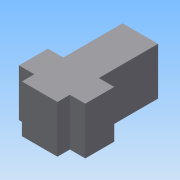
# Autodesk Inventor part: крепеж  для бокса
Saved by Autodesk Inventor 2017 (Build 210142000, 142)
## iProperties
Part Number: крепеж  для бокса
Material: Типовые
Document SubType Name: Modeling
Designer: Max
Mass: 0.64474 g
Surface Area: 6.51926 cm^2
Volume: 0.64474 cm^3
Density: 1 g/cm^3
Appearance: Резина — синяя
Author: Max
Autodesk Inventor part; units mm, degrees
(part 1 of 2)
ref_plane "YZ Plane" through (0, 0, 0) normal (1, 0, 0) x (0, 1, 0)
ref_plane "XZ Plane" through (0, 0, 0) normal (0, 1, 0) x (-1, 0, 0)
ref_plane "XY Plane" through (0, 0, 0) normal (0, 0, 1) x (1, 0, 0)
sketch "Эскиз1" plane through (0, 0, 0) normal (0, 0, 1) x (1, 0, 0)
  line L0 (330.6864, -227.7379) -> (330.6864, -232.7379)
  line L1 (330.6864, -232.7379) -> (331.9864, -232.7379)
  line L2 (331.9864, -232.7379) -> (331.9864, -235.1879)
  line L3 (331.9864, -235.1879) -> (330.6864, -235.1879)
  line L4 (330.6864, -235.1879) -> (330.6864, -236.2379)
  line L5 (330.6864, -236.2379) -> (327.6864, -236.2379)
  line L6 (327.6864, -236.2379) -> (327.6864, -235.1879)
  line L7 (327.6864, -235.1879) -> (326.3864, -235.1879)
  line L8 (326.3864, -235.1879) -> (326.3864, -232.7379)
  line L9 (326.3864, -232.7379) -> (327.6864, -232.7379)
  line L10 (327.6864, -232.7379) -> (327.6864, -227.7379)
  line L11 (327.6864, -227.7379) -> (289.8864, -227.7379)
  line L12 (289.8864, -227.7379) -> (289.8864, -223.7379)
  line L13 (289.8864, -223.7379) -> (212.4864, -223.7379)
  line L14 (212.4864, -223.7379) -> (212.4864, -227.7379)
  line L15 (212.4864, -227.7379) -> (174.8364, -227.7379)
  line L16 (174.8364, -227.7379) -> (174.8364, -232.7379)
  line L17 (174.8364, -232.7379) -> (176.1364, -232.7379)
  line L18 (176.1364, -232.7379) -> (176.1364, -235.1879)
  line L19 (176.1364, -235.1879) -> (174.8364, -235.1879)
  line L20 (174.8364, -235.1879) -> (174.8364, -236.2379)
  line L21 (174.8364, -236.2379) -> (171.8364, -236.2379)
  line L22 (171.8364, -236.2379) -> (171.8364, -235.1879)
  line L23 (171.8364, -235.1879) -> (170.5364, -235.1879)
  line L24 (170.5364, -235.1879) -> (170.5364, -232.7379)
  line L25 (170.5364, -232.7379) -> (171.8364, -232.7379)
  line L26 (171.8364, -232.7379) -> (171.8364, -227.7379)
  line L27 (171.8364, -227.7379) -> (134.1864, -227.7379)
  line L28 (134.1864, -227.7379) -> (134.1864, -735.7379) projected
  line L29 (134.1864, -735.7379) -> (184.1864, -735.7379) projected
  line L30 (184.1864, -735.7379) -> (184.1864, -437.7379) projected
  line L31 (184.1864, -437.7379) -> (204.1864, -417.7379)
  line L32 (204.1864, -417.7379) -> (454.1864, -417.7379)
  line L33 (454.1864, -417.7379) -> (474.1864, -437.7379)
  line L34 (474.1864, -437.7379) -> (474.1864, -735.7379) projected
  line L35 (474.1864, -735.7379) -> (524.1864, -735.7379) projected
  line L36 (524.1864, -735.7379) -> (524.1864, -227.7379) projected
  line L37 (524.1864, -227.7379) -> (486.5364, -227.7379)
  line L38 (486.5364, -227.7379) -> (486.5364, -232.7379)
  line L39 (486.5364, -232.7379) -> (487.8364, -232.7379)
  line L40 (487.8364, -232.7379) -> (487.8364, -235.1879)
  line L41 (487.8364, -235.1879) -> (486.5364, -235.1879)
  line L42 (486.5364, -235.1879) -> (486.5364, -236.2379)
  line L43 (486.5364, -236.2379) -> (483.5364, -236.2379)
  line L44 (483.5364, -236.2379) -> (483.5364, -235.1879)
  line L45 (483.5364, -235.1879) -> (482.2364, -235.1879)
  line L46 (482.2364, -235.1879) -> (482.2364, -232.7379)
  line L47 (482.2364, -232.7379) -> (483.5364, -232.7379)
  line L48 (483.5364, -232.7379) -> (483.5364, -227.7379)
  line L49 (483.5364, -227.7379) -> (445.8864, -227.7379)
  line L50 (445.8864, -227.7379) -> (445.8864, -223.7379)
  line L51 (445.8864, -223.7379) -> (368.4864, -223.7379)
  line L52 (368.4864, -223.7379) -> (368.4864, -227.7379)
  line L53 (368.4864, -227.7379) -> (330.6864, -227.7379)
  circle A0 centre (510.1864, -385.7379) radius 5
  circle A1 centre (148.1864, -385.7379) radius 5
  circle A2 centre (150.1864, -412.7379) radius 5
  circle A3 centre (508.1864, -412.7379) radius 5
  line L54 (198.0365, -283.9874) -> (198.0365, -274.4874)
  arc A4 (198.2865, -274.2374) -> (198.0365, -274.4874) centre (198.2865, -274.4874) ccw
  line L55 (198.2865, -274.2374) -> (220.2865, -274.2374)
  arc A5 (220.5365, -274.4874) -> (220.2865, -274.2374) centre (220.2865, -274.4874) ccw
  line L56 (220.5365, -274.4874) -> (220.5365, -283.9874)
  arc A6 (220.2865, -284.2374) -> (220.5365, -283.9874) centre (220.2865, -283.9874) ccw
  line L57 (220.2865, -284.2374) -> (198.2865, -284.2374)
  arc A7 (198.0365, -283.9874) -> (198.2865, -284.2374) centre (198.2865, -283.9874) ccw
  spline S0 degree 4 poles (220.5005, -310.507) (220.5003, -310.0397) (220.4543, -309.4219) (220.3063, -308.6946) (219.9828, -307.9126) (219.5846, -307.2407) (219.1485, -306.7849) (218.7486, -306.4926) (218.4341, -306.3133) knots 0 0 0 0 0 0.333261 0.458786 0.580687 0.70052 1 1 1 1 1
  spline S1 degree 4 poles (218.4341, -306.3133) (218.2194, -306.2045) (217.9574, -306.0638) (217.2245, -305.8515) (216.8112, -305.759) (215.0952, -305.8521) (214.8239, -305.815) knots 0 0 0 0 0 0.331948 0.48487 1 1 1 1 1
  line L58 (214.8239, -305.815) -> (210.9827, -305.815)
  line L59 (210.9827, -305.815) -> (210.9827, -303.0192)
  line L60 (210.9827, -303.0192) -> (215.6262, -303.0192)
  spline S2 degree 4 poles (215.6262, -303.0192) (216.0632, -302.9791) (218.3041, -303.1205) (219.1074, -303.2602) (220.3376, -303.6977) (220.8048, -303.9727) (221.1813, -304.1983) knots 0 0 0 0 0 0.48869 0.646796 1 1 1 1 1
  spline S3 degree 4 poles (221.1813, -304.1983) (221.6328, -304.4905) (222.2206, -304.9662) (222.87, -305.6808) (223.5166, -306.727) (224.0456, -307.8865) (224.2868, -308.9631) (224.3652, -309.8569) (224.366, -310.5313) knots 0 0 0 0 0 0.30127 0.423004 0.546367 0.672176 1 1 1 1 1
  spline S4 degree 4 poles (224.366, -310.5313) (224.3672, -311.1836) (224.2819, -312.0637) (224.0275, -313.128) (223.4629, -314.3083) (222.7851, -315.3791) (222.1412, -316.0885) (221.5656, -316.5539) (221.1326, -316.8279) knots 0 0 0 0 0 0.325829 0.453052 0.578284 0.70143 1 1 1 1 1
  spline S5 degree 4 poles (221.1326, -316.8279) (220.7893, -317.0305) (220.3484, -317.2658) (219.1646, -317.6777) (218.3558, -317.7448) (216.0857, -318.1145) (215.6748, -318.0192) knots 0 0 0 0 0 0.345082 0.503845 1 1 1 1 1
  line L61 (215.6748, -318.0192) -> (210.9827, -318.0192)
  line L62 (210.9827, -318.0192) -> (210.9827, -315.2112)
  line L63 (210.9827, -315.2112) -> (214.8239, -315.2112)
  spline S6 degree 4 poles (214.8239, -315.2112) (215.1741, -315.246) (216.9237, -315.0068) (217.3918, -315.0434) (218.1403, -314.8454) (218.4072, -314.7315) (218.6164, -314.6278) knots 0 0 0 0 0 0.523746 0.675711 1 1 1 1 1
  spline S7 degree 4 poles (218.6164, -314.6278) (218.8947, -314.4519) (219.2518, -314.164) (219.6429, -313.721) (220.0126, -313.068) (220.3184, -312.3077) (220.4565, -311.5867) (220.5004, -310.9747) (220.5005, -310.507) knots 0 0 0 0 0 0.293933 0.413176 0.535292 0.661734 1 1 1 1 1
  line L64 (206.7865, -285.7374) -> (206.7865, -284.7374)
  line L65 (206.7865, -284.7374) -> (211.7865, -284.7374)
  line L66 (211.7865, -284.7374) -> (211.7865, -285.7374)
  line L67 (211.7865, -285.7374) -> (213.7865, -285.7374)
  line L68 (213.7865, -285.7374) -> (213.7865, -288.7374)
  spline S8 degree 4 poles (213.7865, -288.7374) (213.6519, -288.8139) (213.4737, -288.7819) (213.3015, -288.643) (213.0567, -288.4771) (212.69, -288.3556) (212.2603, -288.4723) (211.871, -288.6284) (211.5365, -288.7374) knots 0 0 0 0 0 0.262205 0.367936 0.481015 0.607227 1 1 1 1 1
  spline S9 degree 4 poles (211.5365, -288.7374) (211.1505, -288.9432) (210.6435, -289.1648) (210.0259, -289.3413) (209.2886, -289.3933) (208.5507, -289.3412) (207.9319, -289.1646) (207.4237, -288.9431) (207.0365, -288.7374) knots 0 0 0 0 0 0.321352 0.440904 0.558717 0.678328 1 1 1 1 1
  spline S10 degree 4 poles (207.0365, -288.7374) (206.8474, -288.9124) (206.596, -289.091) (206.2892, -289.2192) (205.9233, -289.2608) (205.553, -289.2318) (205.2381, -289.1011) (204.981, -288.9152) (204.7865, -288.7374) knots 0 0 0 0 0 0.325734 0.441296 0.554264 0.670467 1 1 1 1 1
  line L69 (204.7865, -288.7374) -> (204.7865, -285.7374)
  line L70 (204.7865, -285.7374) -> (206.7865, -285.7374)
  line L71 (209.6615, -293.1605) -> (208.9115, -293.1605)
  line L72 (208.9115, -293.1605) -> (205.8815, -289.9115)
  spline S11 degree 4 poles (205.8815, -289.9115) (205.9805, -289.9087) (206.1201, -289.8928) (206.2986, -289.8511) (206.5123, -289.7699) (206.7297, -289.6659) (206.9037, -289.5566) (207.0382, -289.4574) (207.1348, -289.3787) knots 0 0 0 0 0 0.300687 0.4228 0.546613 0.672716 1 1 1 1 1
  spline S12 degree 4 poles (207.1348, -289.3787) (207.4869, -289.5458) (207.9624, -289.7299) (208.5607, -289.88) (209.2865, -289.9251) (210.0123, -289.88) (210.6106, -289.7298) (211.0863, -289.5458) (211.4383, -289.3787) knots 0 0 0 0 0 0.318028 0.439699 0.56029 0.681964 1 1 1 1 1
  spline S13 degree 4 poles (211.4383, -289.3787) (211.5621, -289.4198) (211.726, -289.4782) (211.9234, -289.5547) (212.1488, -289.6486) (212.3519, -289.7369) (212.5071, -289.8094) (212.6189, -289.8675) (212.6916, -289.9115) knots 0 0 0 0 0 0.337221 0.465736 0.590517 0.711668 1 1 1 1 1
  line L73 (212.6916, -289.9115) -> (209.6615, -293.1605)
  line L74 (214.751, -315.1701) -> (210.9827, -315.1701)
  line L75 (210.9827, -315.1701) -> (210.9827, -305.8193)
  line L76 (210.9827, -305.8193) -> (214.751, -305.8193)
  line L77 (214.751, -305.8193) -> (214.751, -315.1701)
  arc A8 (209.7865, -300.4106) -> (208.2865, -298.9106) centre (208.2865, -300.4106) ccw
  line L78 (209.7865, -300.4106) -> (209.7865, -300.9106)
  line L79 (209.7865, -300.9106) -> (208.7865, -300.9106)
  line L80 (208.7865, -300.9106) -> (208.7865, -300.4106)
  arc A9 (208.7865, -300.4106) -> (208.2865, -299.9106) centre (208.2865, -300.4106) ccw
  line L81 (208.2865, -299.9106) -> (201.7865, -299.9106)
  arc A10 (201.7865, -296.9106) -> (201.7865, -299.9106) centre (201.7865, -298.4106) ccw
  line L82 (201.7865, -296.9106) -> (216.7865, -296.9106)
  arc A11 (216.7865, -296.9106) -> (216.7865, -295.9106) centre (216.7865, -296.4106) ccw
  line L83 (216.7865, -295.9106) -> (210.2865, -295.9106)
  arc A12 (208.7865, -294.4106) -> (210.2865, -295.9106) centre (210.2865, -294.4106) ccw
  line L84 (208.7865, -294.4106) -> (208.7865, -293.9106)
  line L85 (208.7865, -293.9106) -> (209.7865, -293.9106)
  line L86 (209.7865, -293.9106) -> (209.7865, -294.4106)
  arc A13 (209.7865, -294.4106) -> (210.2865, -294.9106) centre (210.2865, -294.4106) ccw
  line L87 (210.2865, -294.9106) -> (216.7865, -294.9106)
  arc A14 (216.7865, -297.9106) -> (216.7865, -294.9106) centre (216.7865, -296.4106) ccw
  line L88 (216.7865, -297.9106) -> (201.7865, -297.9106)
  arc A15 (201.7865, -297.9106) -> (201.7865, -298.9106) centre (201.7865, -298.4106) ccw
  line L89 (201.7865, -298.9106) -> (208.2865, -298.9106)
  spline S14 degree 4 poles (206.5338, -303.6148) (206.7685, -303.7597) (207.0659, -303.9867) (207.3902, -304.3236) (207.6872, -304.8028) (207.9226, -305.3279) (208.031, -305.7914) (208.0657, -306.1761) (208.0654, -306.4592) knots 0 0 0 0 0 0.312949 0.435922 0.558791 0.682637 1 1 1 1 1
  spline S15 degree 4 poles (208.0654, -306.4592) (208.0667, -306.8455) (207.9969, -307.373) (207.7865, -307.9991) (207.3334, -308.6976) (206.7816, -309.3133) (206.2308, -309.6699) (205.74, -309.8607) (205.3668, -309.9479) knots 0 0 0 0 0 0.313918 0.438715 0.563217 0.687663 1 1 1 1 1
  line L90 (205.3668, -309.9479) -> (205.3668, -310.0937)
  spline S16 degree 4 poles (205.3668, -310.0937) (205.5312, -310.0712) (206.2732, -310.3709) (206.5855, -310.4525) (207.0618, -310.7261) (207.2515, -310.8673) (207.409, -310.9933) knots 0 0 0 0 0 0.467412 0.627499 1 1 1 1 1
  spline S17 degree 4 poles (207.409, -310.9933) (207.5481, -311.1133) (207.7331, -311.307) (207.9398, -311.5886) (208.1607, -311.9975) (208.3429, -312.4401) (208.4267, -312.8625) (208.4538, -313.2077) (208.4544, -313.473) knots 0 0 0 0 0 0.293401 0.414689 0.538726 0.665972 1 1 1 1 1
  spline S18 degree 4 poles (208.4544, -313.473) (208.4542, -313.8182) (208.4167, -314.2867) (208.3007, -314.8566) (208.0496, -315.5046) (207.7363, -316.1003) (207.4002, -316.53) (207.0921, -316.8283) (206.8498, -317.0224) knots 0 0 0 0 0 0.321122 0.446176 0.569734 0.692519 1 1 1 1 1
  spline S19 degree 4 poles (206.8498, -317.0224) (206.6091, -317.215) (206.2427, -317.4621) (205.7289, -317.7312) (205.0243, -317.9925) (204.2362, -318.2079) (203.4791, -318.3046) (202.8516, -318.3351) (202.3644, -318.3352) knots 0 0 0 0 0 0.288505 0.407246 0.52959 0.656869 1 1 1 1 1
  spline S20 degree 4 poles (202.3644, -318.3352) (200.7651, -318.3047) (199.5638, -318.1496) (198.2039, -317.74) (197.3198, -317.3871) knots 0 0 0 0 0 1 1 1 1 1
  line L91 (197.3198, -317.3871) -> (197.3198, -314.1294)
  line L92 (197.3198, -314.1294) -> (197.6845, -314.1294)
  spline S21 degree 4 poles (197.6845, -314.1294) (197.8963, -314.3375) (199.3348, -314.8985) (200.0458, -315.1512) (200.9862, -315.3661) (201.3735, -315.4088) (201.6594, -315.43) knots 0 0 0 0 0 0.485606 0.650571 1 1 1 1 1
  spline S22 degree 4 poles (201.6594, -315.43) (201.8017, -315.4566) (202.7287, -315.3618) (203.1091, -315.3075) (203.6053, -315.1248) (203.7864, -315.012) (203.9203, -314.9195) knots 0 0 0 0 0 0.490597 0.653392 1 1 1 1 1
  spline S23 degree 4 poles (203.9203, -314.9195) (204.0251, -314.8403) (204.1632, -314.7177) (204.3146, -314.5417) (204.4732, -314.2933) (204.5993, -314.0182) (204.6569, -313.7148) (204.6734, -313.4623) (204.674, -313.2542) knots 0 0 0 0 0 0.293695 0.410721 0.530018 0.654429 1 1 1 1 1
  spline S24 degree 4 poles (204.674, -313.2542) (204.6737, -313.05) (204.65, -312.7949) (204.5704, -312.5) (204.3941, -312.2275) (204.1685, -311.9914) (203.9524, -311.8427) (203.754, -311.7508) (203.6043, -311.6983) knots 0 0 0 0 0 0.332874 0.455336 0.574642 0.693712 1 1 1 1 1
  spline S25 degree 3 poles (203.6043, -311.6983) (203.1339, -311.419) (202.8478, -311.2752) (201.2461, -311.4916) knots 0 0 0 0 1 1 1 1
  line L93 (201.2461, -311.4916) -> (200.6018, -311.4916)
  line L94 (200.6018, -311.4916) -> (200.6018, -308.8539)
  line L95 (200.6018, -308.8539) -> (201.1975, -308.8539)
  spline S26 degree 4 poles (201.1975, -308.8539) (201.8646, -308.8347) (202.5816, -308.7738) (203.0974, -308.7347) (203.4341, -308.55) knots 0 0 0 0 0 1 1 1 1 1
  spline S27 degree 4 poles (203.4341, -308.55) (203.5568, -308.4899) (203.7161, -308.3919) (203.8905, -308.2415) (204.0639, -308.0177) (204.2017, -307.7644) (204.265, -307.4981) (204.2843, -307.2719) (204.285, -307.0913) knots 0 0 0 0 0 0.303428 0.422137 0.541736 0.664935 1 1 1 1 1
  spline S28 degree 4 poles (204.285, -307.0913) (204.2846, -306.9506) (204.2677, -306.7719) (204.2092, -306.5582) (204.0845, -306.3506) (203.9226, -306.1579) (203.7804, -306.033) (203.6505, -305.9492) (203.5557, -305.9001) knots 0 0 0 0 0 0.328861 0.453441 0.575803 0.697309 1 1 1 1 1
  spline S29 degree 4 poles (203.5557, -305.9001) (203.4448, -305.8495) (203.2969, -305.7896) (202.9114, -305.6871) (202.6272, -305.6603) (201.9555, -305.5746) (201.8782, -305.5962) knots 0 0 0 0 0 0.352064 0.518119 1 1 1 1 1
  spline S30 degree 4 poles (201.8782, -305.5962) (201.3241, -305.5966) (200.7829, -305.6848) (200.1681, -305.8558) (199.6416, -306.0581) knots 0 0 0 0 0 1 1 1 1 1
  spline S31 degree 3 poles (199.6416, -306.0581) (200.0559, -305.6978) (203.2118, -303.6988) (198.2887, -306.7332) knots 0 0 0 0 1 1 1 1
  line L96 (198.2887, -306.7332) -> (197.8235, -306.8604)
  line L97 (197.8235, -306.8604) -> (197.7574, -306.8604)
  line L98 (197.7574, -306.8604) -> (197.7574, -303.6513)
  spline S32 degree 4 poles (197.7574, -303.6513) (198.6005, -303.3178) (200.0612, -302.9118) (201.2135, -302.7136) (202.5346, -302.7031) knots 0 0 0 0 0 1 1 1 1 1
  spline S33 degree 4 poles (202.5346, -302.7031) (203.7734, -302.7074) (204.8441, -302.8363) (205.7919, -303.1378) (206.5338, -303.6148) knots 0 0 0 0 0 1 1 1 1 1
  line L99 (209.1913, -331.2373) -> (209.1913, -324.7373)
  arc A16 (209.1913, -324.7373) -> (209.1912, -324.7373) centre (209.2865, -297.2374) ccw
  line L100 (209.1912, -324.7373) -> (209.1912, -331.2373)
  arc A17 (204.7865, -330.9383) -> (209.1912, -331.2373) centre (209.2865, -297.2374) ccw
  arc A18 (203.0365, -327.6009) -> (204.7865, -330.9383) centre (216.5671, -322.6337) ccw
  arc A19 (192.2358, -323.127) -> (203.0365, -327.6009) centre (209.2865, -297.2374) ccw
  arc A20 (188.6384, -324.2495) -> (192.2358, -323.127) centre (186.1806, -310.0472) ccw
  arc A21 (182.2744, -317.8856) -> (188.6384, -324.2495) centre (209.2865, -297.2374) ccw
  arc A22 (183.3969, -314.2882) -> (182.2744, -317.8856) centre (196.4768, -320.3434) ccw
  arc A23 (178.9231, -303.4874) -> (183.3969, -314.2882) centre (209.2865, -297.2374) ccw
  arc A24 (175.5856, -301.7374) -> (178.9231, -303.4874) centre (183.8903, -289.9569) ccw
  arc A25 (175.5856, -292.7374) -> (175.5856, -301.7374) centre (209.2865, -297.2374) ccw
  arc A26 (178.9231, -290.9874) -> (175.5856, -292.7374) centre (183.8903, -304.518) ccw
  arc A27 (183.3969, -280.1867) -> (178.9231, -290.9874) centre (209.2865, -297.2374) ccw
  arc A28 (182.2744, -276.5893) -> (183.3969, -280.1867) centre (196.4768, -274.1315) ccw
  arc A29 (188.6384, -270.2253) -> (182.2744, -276.5893) centre (209.2865, -297.2374) ccw
  arc A30 (192.2358, -271.3478) -> (188.6384, -270.2253) centre (186.1806, -284.4277) ccw
  arc A31 (203.0365, -266.874) -> (192.2358, -271.3478) centre (209.2865, -297.2374) ccw
  arc A32 (204.7865, -263.5365) -> (203.0365, -266.874) centre (216.5671, -271.8412) ccw
  arc A33 (213.7865, -263.5365) -> (204.7865, -263.5365) centre (209.2865, -297.2374) ccw
  arc A34 (215.5365, -266.874) -> (213.7865, -263.5365) centre (202.006, -271.8412) ccw
  arc A35 (226.3373, -271.3478) -> (215.5365, -266.874) centre (209.2865, -297.2374) ccw
  arc A36 (229.9347, -270.2253) -> (226.3373, -271.3478) centre (232.3925, -284.4277) ccw
  arc A37 (236.2986, -276.5893) -> (229.9347, -270.2253) centre (209.2865, -297.2374) ccw
  arc A38 (235.1761, -280.1867) -> (236.2986, -276.5893) centre (222.0963, -274.1315) ccw
  arc A39 (239.65, -290.9874) -> (235.1761, -280.1867) centre (209.2865, -297.2374) ccw
  arc A40 (242.9874, -292.7374) -> (239.65, -290.9874) centre (234.6828, -304.518) ccw
  arc A41 (242.9874, -301.7374) -> (242.9874, -292.7374) centre (209.2865, -297.2374) ccw
  arc A42 (239.65, -303.4874) -> (242.9874, -301.7374) centre (234.6828, -289.9569) ccw
  arc A43 (235.1761, -314.2882) -> (239.65, -303.4874) centre (209.2865, -297.2374) ccw
  arc A44 (236.2986, -317.8856) -> (235.1761, -314.2882) centre (222.0963, -320.3434) ccw
  arc A45 (229.9347, -324.2495) -> (236.2986, -317.8856) centre (209.2865, -297.2374) ccw
  arc A46 (226.3373, -323.127) -> (229.9347, -324.2495) centre (232.3925, -310.0472) ccw
  arc A47 (215.5365, -327.6009) -> (226.3373, -323.127) centre (209.2865, -297.2374) ccw
  arc A48 (213.7865, -330.9383) -> (215.5365, -327.6009) centre (202.006, -322.6337) ccw
  arc A49 (209.1913, -331.2373) -> (213.7865, -330.9383) centre (209.2865, -297.2374) ccw
  circle A50 centre (330.1864, -297.7379) radius 20.6
  circle A51 centre (508.6864, -721.7379) radius 2 projected
  circle A52 centre (149.6864, -682.2379) radius 2 projected
  circle A53 centre (149.6864, -424.7379) radius 2
  circle A54 centre (508.6864, -424.7379) radius 2
  circle A55 centre (508.6864, -506.7379) radius 2.875 projected
  circle A56 centre (149.6864, -453.7379) radius 2
  circle A57 centre (149.6864, -721.7379) radius 2 projected
  circle A58 centre (170.4364, -639.7379) radius 1.5 projected
  circle A59 centre (170.4364, -507.7379) radius 1.5 projected
  circle A60 centre (170.4364, -477.7379) radius 1.5
  circle A61 centre (170.4364, -669.7379) radius 1.5 projected
  circle A62 centre (479.4534, -583.2596) radius 1.5 projected
  line L101 (445.4108, -378.2955) -> (445.4108, -381.1733)
  line L102 (445.4108, -381.1733) -> (439.6177, -381.1733)
  line L103 (439.6177, -381.1733) -> (439.3174, -383.1252)
  spline S34 degree 4 poles (439.3174, -383.1252) (439.8832, -382.9763) (440.4727, -382.8362) (441.0568, -382.6943) (441.6697, -382.5621) knots 0 0 0 0 0 1 1 1 1 1
  spline S35 degree 4 poles (441.6697, -382.5621) (442.2638, -382.5598) (443.052, -382.6679) (443.9476, -382.9985) (444.8569, -383.7336) (445.5947, -384.609) (445.9315, -385.4454) (446.0393, -386.1746) (446.0364, -386.7161) knots 0 0 0 0 0 0.321 0.445325 0.568168 0.690637 1 1 1 1 1
  spline S36 degree 4 poles (446.0364, -386.7161) (446.0346, -387.3159) (445.9109, -388.0809) (445.4981, -389.1528) (444.7052, -390.1668) (443.6543, -391.0177) (442.5576, -391.4124) (441.5087, -391.5161) (440.7063, -391.5207) knots 0 0 0 0 0 0.301808 0.422596 0.543783 0.666952 1 1 1 1 1
  spline S37 degree 4 poles (440.7063, -391.5207) (439.918, -391.5188) (438.9727, -391.4394) (437.9148, -391.1682) (436.9202, -390.5588) (436.1038, -389.8278) (435.6627, -389.1519) (435.3981, -388.4698) (435.2385, -387.9298) knots 0 0 0 0 0 0.344288 0.467767 0.585513 0.701061 1 1 1 1 1
  line L104 (435.2385, -387.9298) -> (438.892, -387.5294)
  spline S38 degree 4 poles (438.892, -387.5294) (438.9412, -387.7989) (439.0435, -388.1412) (439.2278, -388.5159) (439.5476, -388.8668) (439.8937, -389.136) (440.207, -389.2665) (440.4728, -389.3137) (440.6687, -389.3186) knots 0 0 0 0 0 0.337823 0.463732 0.585419 0.704571 1 1 1 1 1
  spline S39 degree 4 poles (440.6687, -389.3186) (440.8901, -389.3188) (441.1893, -389.2693) (441.5319, -389.1156) (441.8931, -388.7807) (442.2105, -388.3375) (442.349, -387.842) (442.3952, -387.3979) (442.3954, -387.0414) knots 0 0 0 0 0 0.288865 0.405011 0.524609 0.650411 1 1 1 1 1
  spline S40 degree 4 poles (442.3954, -387.0414) (442.3965, -386.6796) (442.3506, -386.2306) (442.2143, -385.7358) (441.8934, -385.3038) (441.5184, -384.9825) (441.1547, -384.8384) (440.8338, -384.7976) (440.5936, -384.8018) knots 0 0 0 0 0 0.347295 0.471219 0.589277 0.705046 1 1 1 1 1
  spline S41 degree 4 poles (440.5936, -384.8018) (440.3308, -384.8028) (440.0722, -384.8472) (439.8214, -384.9358) (439.5802, -385.0645) knots 0 0 0 0 0 1 1 1 1 1
  spline S42 degree 4 poles (439.5802, -385.0645) (439.4113, -385.0419) (439.2106, -385.2032) (439.0118, -385.4464) (438.7919, -385.7277) knots 0 0 0 0 0 1 1 1 1 1
  line L105 (438.7919, -385.7277) -> (435.714, -385.2897)
  line L106 (435.714, -385.2897) -> (436.8526, -378.2955)
  line L107 (436.8526, -378.2955) -> (445.4108, -378.2955)
  spline S43 degree 4 poles (406.7861, -386.7537) (406.783, -386.8994) (406.9374, -387.4742) (407.0204, -387.7031) (407.1624, -387.996) (407.2325, -388.1023) (407.2866, -388.18) knots 0 0 0 0 0 0.506296 0.664932 1 1 1 1 1
  spline S44 degree 4 poles (407.2866, -388.18) (407.382, -388.3002) (407.5282, -388.4525) (407.7394, -388.6182) (408.0321, -388.7711) (408.3561, -388.8938) (408.6492, -388.9503) (408.8932, -388.9682) (409.0758, -388.9683) knots 0 0 0 0 0 0.304407 0.425791 0.548382 0.673395 1 1 1 1 1
  spline S45 degree 4 poles (409.0758, -388.9683) (409.3418, -388.9666) (409.6834, -388.9198) (410.0596, -388.803) (410.4185, -388.5341) (410.6892, -388.2467) (410.8181, -387.9944) (410.8631, -387.7819) (410.8651, -387.6295) knots 0 0 0 0 0 0.349494 0.478462 0.601477 0.719585 1 1 1 1 1
  spline S46 degree 4 poles (410.8651, -387.6295) (410.8651, -387.5535) (410.8554, -387.4485) (410.8248, -387.3165) (410.7593, -387.1612) (410.6716, -387.0048) (410.5753, -386.883) (410.4859, -386.792) (410.4146, -386.7286) knots 0 0 0 0 0 0.300852 0.421911 0.544763 0.670489 1 1 1 1 1
  spline S47 degree 4 poles (410.4146, -386.7286) (410.1571, -386.5044) (409.6674, -386.3111) (409.0725, -386.1312) (408.3627, -385.9654) knots 0 0 0 0 0 1 1 1 1 1
  spline S48 degree 4 poles (408.3627, -385.9654) (407.1494, -385.6938) (406.0889, -385.3543) (405.2024, -384.9288) (404.584, -384.3889) knots 0 0 0 0 0 1 1 1 1 1
  spline S49 degree 4 poles (404.584, -384.3889) (404.408, -384.2361) (404.1857, -384.0093) (403.9447, -383.6933) (403.7233, -383.2707) (403.5506, -382.824) (403.4707, -382.4311) (403.4454, -382.1105) (403.4454, -381.874) knots 0 0 0 0 0 0.314239 0.437484 0.560343 0.683894 1 1 1 1 1
  spline S50 degree 4 poles (403.4454, -381.874) (403.4449, -381.4151) (403.5577, -380.8163) (403.9167, -380.0101) (404.6502, -379.2264) (405.7309, -378.5045) (406.8706, -378.1485) (408.0596, -378.0831) (408.9757, -378.0703) knots 0 0 0 0 0 0.276596 0.390848 0.509627 0.635941 1 1 1 1 1
  spline S51 degree 4 poles (408.9757, -378.0703) (409.7519, -378.0735) (410.7314, -378.1522) (411.8268, -378.4191) (412.8553, -379.0125) (413.6516, -379.7584) (414.0771, -380.5932) (414.2667, -381.3518) (414.3434, -381.949) knots 0 0 0 0 0 0.340632 0.462675 0.579541 0.695373 1 1 1 1 1
  line L108 (414.3434, -381.949) -> (410.5523, -382.1743)
  spline S52 degree 4 poles (410.5523, -382.1743) (410.5026, -381.9089) (410.4058, -381.5777) (410.2218, -381.2167) (409.9086, -380.8975) (409.5367, -380.6514) (409.1622, -380.5366) (408.8314, -380.5001) (408.5754, -380.4976) knots 0 0 0 0 0 0.324684 0.444588 0.562205 0.68129 1 1 1 1 1
  spline S53 degree 4 poles (408.5754, -380.4976) (408.3547, -380.4984) (408.0765, -380.531) (407.7733, -380.6151) (407.4955, -380.8115) (407.2908, -381.0256) (407.1945, -381.225) (407.1626, -381.397) (407.1615, -381.5236) knots 0 0 0 0 0 0.354168 0.481315 0.601534 0.717295 1 1 1 1 1
  spline S54 degree 4 poles (407.1615, -381.5236) (407.151, -381.5513) (407.1425, -381.5923) (407.1555, -381.6537) (407.1952, -381.7382) (407.2603, -381.845) (407.3352, -381.9396) (407.4052, -382.0169) (407.4618, -382.0742) knots 0 0 0 0 0 0.247386 0.359721 0.483602 0.619276 1 1 1 1 1
  spline S55 degree 4 poles (407.4618, -382.0742) (407.502, -382.1096) (407.5742, -382.1593) (407.6951, -382.2227) (407.9699, -382.3345) (408.225, -382.4111) (408.4138, -382.46) (408.8131, -382.5496) knots 0 0 0 0 0 0.265093 0.389381 0.526504 1 1 1 1 1
  spline S56 degree 4 poles (408.8131, -382.5496) (409.9591, -382.8033) (411.5127, -383.2002) (412.6708, -383.6431) (413.7254, -384.4472) (414.3811, -385.2229) (414.6765, -385.9927) (414.7705, -386.6006) (414.7688, -387.0665) knots 0 0 0 0 0 0.389595 0.513425 0.625734 0.733468 1 1 1 1 1
  spline S57 degree 4 poles (414.7688, -387.0665) (414.7651, -387.6424) (414.6429, -388.3842) (414.1942, -389.3533) (413.3387, -390.2809) (412.195, -391.0651) (411.0021, -391.4207) (409.8737, -391.5173) (409.0008, -391.5207) knots 0 0 0 0 0 0.292777 0.410851 0.531211 0.655943 1 1 1 1 1
  spline S58 degree 4 poles (409.0008, -391.5207) (407.9895, -391.5206) (406.7811, -391.4067) (405.4293, -391.0713) (404.3652, -390.2519) (403.5782, -389.2777) (403.1749, -388.3819) (403.0083, -387.5819) (402.9575, -386.9914) knots 0 0 0 0 0 0.35491 0.478284 0.59487 0.709037 1 1 1 1 1
  line L109 (402.9575, -386.9914) -> (406.7861, -386.7537)
  spline S59 degree 4 poles (394.7371, -378.0703) (395.7191, -378.07) (396.9898, -378.2189) (398.4153, -378.6999) (399.7793, -379.7808) (400.8604, -381.1289) (401.3447, -382.5175) (401.4939, -383.753) (401.4936, -384.7017) knots 0 0 0 0 0 0.321996 0.442966 0.562085 0.682373 1 1 1 1 1
  spline S60 degree 4 poles (401.4936, -384.7017) (401.4851, -385.7192) (401.3652, -387.0404) (400.8679, -388.4392) (399.8128, -389.7826) (398.4904, -390.8562) (397.1164, -391.3853) (395.8566, -391.5119) (394.8872, -391.5207) knots 0 0 0 0 0 0.324201 0.444012 0.561748 0.68112 1 1 1 1 1
  spline S61 degree 4 poles (394.8872, -391.5207) (393.9051, -391.5237) (392.6153, -391.3825) (391.2354, -390.9616) (389.8902, -389.9369) (388.7595, -388.5767) (388.1566, -387.1369) (388.0342, -385.8227) (388.0181, -384.8018) knots 0 0 0 0 0 0.317732 0.436395 0.554274 0.675018 1 1 1 1 1
  spline S62 degree 4 poles (388.0181, -384.8018) (388.017, -383.8398) (388.1688, -382.5871) (388.6587, -381.1773) (389.7545, -379.8084) (391.1224, -378.7124) (392.5286, -378.2217) (393.7783, -378.0695) (394.7371, -378.0703) knots 0 0 0 0 0 0.319418 0.440426 0.560018 0.68097 1 1 1 1 1
  line L110 (364.7958, -383.8884) -> (371.0017, -383.8884)
  line L111 (371.0017, -383.8884) -> (371.0017, -389.4187)
  spline S63 degree 4 poles (371.0017, -389.4187) (369.2773, -390.5761) (367.9432, -391.1503) (366.483, -391.341) (364.5956, -391.5207) knots 0 0 0 0 0 1 1 1 1 1
  spline S64 degree 4 poles (364.5956, -391.5207) (363.5663, -391.5174) (362.2259, -391.3822) (360.8136, -390.891) (359.4739, -389.7879) (358.4229, -388.4046) (357.8973, -386.926) (357.756, -385.7341) (357.7515, -384.7893) knots 0 0 0 0 0 0.324055 0.444084 0.562865 0.683419 1 1 1 1 1
  spline S65 degree 4 poles (357.7515, -384.7893) (357.7514, -384.1263) (357.8305, -383.2389) (358.08, -382.1878) (358.6262, -381.0385) (359.3014, -380.0325) (360.0273, -379.366) (360.6882, -378.9465) (361.2048, -378.6959) knots 0 0 0 0 0 0.325345 0.450117 0.57259 0.694038 1 1 1 1 1
  spline S66 degree 4 poles (361.2048, -378.6959) (361.9122, -378.363) (362.7618, -378.1622) (363.7151, -378.0709) (364.7582, -378.0703) knots 0 0 0 0 0 1 1 1 1 1
  spline S67 degree 4 poles (364.7582, -378.0703) (365.6777, -378.0749) (366.95, -378.1343) (367.9815, -378.3613) (369.0464, -378.967) (369.8787, -379.6881) (370.3859, -380.4767) (370.6707, -381.1881) (370.8266, -381.7488) knots 0 0 0 0 0 0.355167 0.475286 0.589187 0.703074 1 1 1 1 1
  line L112 (370.8266, -381.7488) -> (366.9478, -382.4495)
  spline S68 degree 4 poles (366.9478, -382.4495) (366.8814, -382.2273) (366.7537, -381.9399) (366.5276, -381.6226) (366.158, -381.3184) (365.7254, -381.0709) (365.3057, -380.9576) (364.9456, -380.9221) (364.6706, -380.923) knots 0 0 0 0 0 0.306162 0.426653 0.548001 0.672045 1 1 1 1 1
  spline S69 degree 4 poles (364.6706, -380.923) (364.2835, -380.9239) (363.7673, -381.0025) (363.1828, -381.2508) (362.5857, -381.7934) (362.0729, -382.5227) (361.8522, -383.3711) (361.781, -384.1317) (361.7804, -384.7517) knots 0 0 0 0 0 0.291183 0.405965 0.523705 0.648116 1 1 1 1 1
  spline S70 degree 4 poles (361.7804, -384.7517) (361.779, -385.4039) (361.8504, -386.201) (362.0651, -387.0776) (362.5841, -387.8163) (363.2003, -388.3522) (363.8218, -388.5952) (364.3751, -388.6679) (364.7958, -388.668) knots 0 0 0 0 0 0.352198 0.4751 0.591203 0.705096 1 1 1 1 1
  spline S71 degree 4 poles (364.7958, -388.668) (365.5044, -388.577) (366.1093, -388.5966) (366.7466, -388.3761) (367.4859, -387.8047) knots 0 0 0 0 0 1 1 1 1 1
  line L113 (367.4859, -387.8047) -> (367.4859, -386.591)
  line L114 (367.4859, -386.591) -> (364.7958, -386.591)
  line L115 (364.7958, -386.591) -> (364.7958, -383.8884)
  line L116 (338.1076, -378.2955) -> (344.8015, -378.2955)
  spline S72 degree 4 poles (344.8015, -378.2955) (345.6091, -378.3087) (346.7113, -378.4377) (347.6525, -378.6374) (348.5774, -379.2274) (349.2936, -379.9502) (349.6937, -380.7224) (349.8093, -381.3789) (349.8314, -381.899) knots 0 0 0 0 0 0.352761 0.473532 0.588688 0.703565 1 1 1 1 1
  spline S73 degree 4 poles (349.8314, -381.899) (349.8301, -382.2318) (349.7876, -382.6715) (349.6583, -383.1996) (349.3774, -383.7638) (349.0247, -384.2843) (348.6726, -384.6428) (348.3514, -384.887) (348.1047, -385.0395) knots 0 0 0 0 0 0.322749 0.447008 0.569667 0.691923 1 1 1 1 1
  spline S74 degree 4 poles (348.1047, -385.0395) (347.8307, -385.2057) (347.496, -385.3436) (347.1142, -385.458) (346.6909, -385.5525) knots 0 0 0 0 0 1 1 1 1 1
  spline S75 degree 4 poles (346.6909, -385.5525) (347.0198, -385.6624) (347.3099, -385.7772) (347.5565, -385.8979) (347.7419, -386.028) knots 0 0 0 0 0 1 1 1 1 1
  spline S76 degree 4 poles (347.7419, -386.028) (347.9857, -386.1912) (348.3728, -386.7098) (348.7642, -387.2731) (348.943, -387.5294) knots 0 0 0 0 0 1 1 1 1 1
  line L117 (348.943, -387.5294) -> (350.8824, -391.2955)
  line L118 (350.8824, -391.2955) -> (346.3405, -391.2955)
  line L119 (346.3405, -391.2955) -> (344.201, -387.3167)
  spline S77 degree 4 poles (344.201, -387.3167) (344.0179, -386.9651) (343.8381, -386.6724) (343.662, -386.4348) (343.4878, -386.3157) knots 0 0 0 0 0 1 1 1 1 1
  spline S78 degree 4 poles (343.4878, -386.3157) (343.4088, -386.2821) (343.2985, -386.2387) (343.1573, -386.1886) (342.9856, -386.1353) (342.8174, -386.0877) (342.6805, -386.054) (342.5746, -386.0307) (342.4993, -386.0154) knots 0 0 0 0 0 0.319421 0.445306 0.570084 0.693867 1 1 1 1 1
  line L120 (342.4993, -386.0154) -> (342.149, -386.0154)
  line L121 (342.149, -386.0154) -> (342.149, -391.2955)
  line L122 (342.149, -391.2955) -> (338.1076, -391.2955)
  line L123 (338.1076, -391.2955) -> (338.1076, -378.2955)
  line L124 (327.3348, -389.1435) -> (326.6966, -391.2955)
  line L125 (326.6966, -391.2955) -> (322.5927, -391.2955)
  line L126 (322.5927, -391.2955) -> (327.4849, -378.2955)
  line L127 (327.4849, -378.2955) -> (331.8766, -378.2955)
  line L128 (331.8766, -378.2955) -> (336.7563, -391.2955)
  line L129 (336.7563, -391.2955) -> (332.5523, -391.2955)
  line L130 (332.5523, -391.2955) -> (331.9016, -389.1435)
  line L131 (331.9016, -389.1435) -> (327.3348, -389.1435)
  spline S79 degree 4 poles (304.175, -378.2955) (304.7349, -378.3254) (305.4521, -378.4569) (306.2431, -378.7599) (307.004, -379.3637) (307.6019, -380.0322) (307.9098, -380.6334) (308.0389, -381.1529) (308.0662, -381.5361) knots 0 0 0 0 0 0.339175 0.465743 0.588018 0.70738 1 1 1 1 1
  spline S80 degree 4 poles (308.0662, -381.5361) (308.0662, -381.7157) (308.0501, -381.9603) (307.9997, -382.2627) (307.8909, -382.6122) (307.7527, -382.9444) (307.6022, -383.1988) (307.4632, -383.3854) (307.353, -383.513) knots 0 0 0 0 0 0.318242 0.442778 0.566311 0.689578 1 1 1 1 1
  spline S81 degree 4 poles (307.353, -383.513) (307.0925, -383.7887) (306.7639, -384.026) (306.377, -384.2252) (305.9392, -384.3889) knots 0 0 0 0 0 1 1 1 1 1
  spline S82 degree 4 poles (305.9392, -384.3889) (306.3709, -384.4933) (306.9124, -384.6821) (307.505, -385.0107) (308.0317, -385.5503) (308.432, -386.1596) (308.6145, -386.7363) (308.6689, -387.232) (308.6668, -387.6045) knots 0 0 0 0 0 0.33021 0.452879 0.572465 0.691726 1 1 1 1 1
  spline S83 degree 4 poles (308.6668, -387.6045) (308.6652, -387.9112) (308.6202, -388.3285) (308.4873, -388.836) (308.2026, -389.4094) (307.8488, -389.9416) (307.4905, -390.3039) (307.1656, -390.5463) (306.9151, -390.6949) knots 0 0 0 0 0 0.316233 0.441052 0.565287 0.689327 1 1 1 1 1
  spline S84 degree 4 poles (306.9151, -390.6949) (306.6369, -390.8493) (306.2765, -390.966) (305.8583, -391.0549) (305.3887, -391.1204) knots 0 0 0 0 0 1 1 1 1 1
  spline S85 degree 2 poles (305.3887, -391.1204) (304.1262, -391.4374) (303.5869, -391.2955) knots 0 0 0 1 1 1
  line L132 (303.5869, -391.2955) -> (296.6553, -391.2955)
  line L133 (296.6553, -391.2955) -> (296.6553, -378.2955)
  line L134 (296.6553, -378.2955) -> (304.175, -378.2955)
  line L135 (264.0864, -378.2955) -> (268.9912, -385.4899)
  line L136 (268.9912, -385.4899) -> (268.9912, -378.2955)
  line L137 (268.9912, -378.2955) -> (272.7823, -378.2955)
  line L138 (272.7823, -378.2955) -> (272.7823, -391.2955)
  line L139 (272.7823, -391.2955) -> (268.9912, -391.2955)
  line L140 (268.9912, -391.2955) -> (264.1115, -384.1386)
  line L141 (264.1115, -384.1386) -> (264.1115, -391.2955)
  line L142 (264.1115, -391.2955) -> (260.3328, -391.2955)
  line L143 (260.3328, -391.2955) -> (260.3328, -378.2955)
  line L144 (260.3328, -378.2955) -> (264.0864, -378.2955)
  line L145 (242.2529, -378.2955) -> (244.868, -382.6747)
  line L146 (244.868, -382.6747) -> (247.4955, -378.2955)
  line L147 (247.4955, -378.2955) -> (251.9373, -378.2955)
  line L148 (251.9373, -378.2955) -> (246.8824, -385.8528)
  line L149 (246.8824, -385.8528) -> (246.8824, -391.2955)
  line L150 (246.8824, -391.2955) -> (242.8535, -391.2955)
  line L151 (242.8535, -391.2955) -> (242.8535, -385.8528)
  line L152 (242.8535, -385.8528) -> (237.7862, -378.2955)
  line L153 (237.7862, -378.2955) -> (242.2529, -378.2955)
  line L154 (224.7987, -378.2955) -> (224.7987, -381.0857)
  line L155 (224.7987, -381.0857) -> (218.918, -381.0857)
  line L156 (218.918, -381.0857) -> (218.918, -383.3504)
  line L157 (218.918, -383.3504) -> (223.9353, -383.3504)
  line L158 (223.9353, -383.3504) -> (223.9353, -385.9779)
  line L159 (223.9353, -385.9779) -> (218.918, -385.9779)
  line L160 (218.918, -385.9779) -> (218.918, -391.2955)
  line L161 (218.918, -391.2955) -> (214.8766, -391.2955)
  line L162 (214.8766, -391.2955) -> (214.8766, -378.2955)
  line L163 (214.8766, -378.2955) -> (224.7987, -378.2955)
  line L164 (230.9921, -378.2955) -> (230.9921, -388.0924)
  line L165 (230.9921, -388.0924) -> (237.2606, -388.0924)
  line L166 (237.2606, -388.0924) -> (237.2606, -391.2955)
  line L167 (237.2606, -391.2955) -> (226.9758, -391.2955)
  line L168 (226.9758, -391.2955) -> (226.9758, -378.2955)
  line L169 (226.9758, -378.2955) -> (230.9921, -378.2955)
  line L170 (257.43, -378.2955) -> (257.43, -391.2955)
  line L171 (257.43, -391.2955) -> (253.4012, -391.2955)
  line L172 (253.4012, -391.2955) -> (253.4012, -378.2955)
  line L173 (253.4012, -378.2955) -> (257.43, -378.2955)
  line L174 (282.0037, -383.8884) -> (288.2096, -383.8884)
  line L175 (288.2096, -383.8884) -> (288.2096, -389.4187)
  spline S86 degree 4 poles (288.2096, -389.4187) (286.4831, -390.5901) (285.1655, -391.2179) (283.6983, -391.3753) (281.8035, -391.5207) knots 0 0 0 0 0 1 1 1 1 1
  spline S87 degree 4 poles (281.8035, -391.5207) (280.7742, -391.5173) (279.4339, -391.3822) (278.0216, -390.8912) (276.6819, -389.7883) (275.631, -388.4051) (275.1054, -386.9264) (274.964, -385.7344) (274.9594, -384.7893) knots 0 0 0 0 0 0.324047 0.444069 0.562844 0.683396 1 1 1 1 1
  spline S88 degree 4 poles (274.9594, -384.7893) (274.9592, -384.1263) (275.0384, -383.2389) (275.2879, -382.1877) (275.8341, -381.0385) (276.5093, -380.0325) (277.2352, -379.366) (277.8961, -378.9465) (278.4127, -378.6959) knots 0 0 0 0 0 0.325346 0.450118 0.572591 0.694038 1 1 1 1 1
  spline S89 degree 4 poles (278.4127, -378.6959) (279.1198, -378.3623) (279.9695, -378.1615) (280.9229, -378.0705) (281.9661, -378.0703) knots 0 0 0 0 0 1 1 1 1 1
  spline S90 degree 4 poles (281.9661, -378.0703) (282.8845, -378.0757) (284.1551, -378.1355) (285.1849, -378.3646) (286.2488, -378.9704) (287.0813, -379.691) (287.5901, -380.4782) (287.8769, -381.1887) (288.0345, -381.7488) knots 0 0 0 0 0 0.355058 0.475172 0.589089 0.703004 1 1 1 1 1
  line L176 (288.0345, -381.7488) -> (284.1557, -382.4495)
  spline S91 degree 4 poles (284.1557, -382.4495) (284.0824, -382.2284) (283.9474, -381.9438) (283.717, -381.6297) (283.3481, -381.3278) (282.9198, -381.0813) (282.5061, -380.9653) (282.1504, -380.9259) (281.8785, -380.923) knots 0 0 0 0 0 0.307304 0.427941 0.549228 0.673035 1 1 1 1 1
  spline S92 degree 4 poles (281.8785, -380.923) (281.491, -380.923) (280.9742, -381) (280.3887, -381.2467) (279.7908, -381.7886) (279.2779, -382.5184) (279.0584, -383.3685) (278.9881, -384.1305) (278.9883, -384.7517) knots 0 0 0 0 0 0.291146 0.405883 0.523583 0.647981 1 1 1 1 1
  spline S93 degree 4 poles (278.9883, -384.7517) (278.9869, -385.4039) (279.0583, -386.201) (279.273, -387.0776) (279.792, -387.8163) (280.4082, -388.3522) (281.0297, -388.5952) (281.583, -388.6679) (282.0037, -388.668) knots 0 0 0 0 0 0.352198 0.475101 0.591203 0.705096 1 1 1 1 1
  spline S94 degree 4 poles (282.0037, -388.668) (282.7126, -388.5709) (283.3158, -388.6011) (283.9561, -388.3869) (284.6938, -387.8047) knots 0 0 0 0 0 1 1 1 1 1
  line L177 (284.6938, -387.8047) -> (284.6938, -386.591)
  line L178 (284.6938, -386.591) -> (282.0037, -386.591)
  line L179 (282.0037, -386.591) -> (282.0037, -383.8884)
  line L180 (321.5417, -378.2955) -> (321.5417, -381.0732)
  line L181 (321.5417, -381.0732) -> (314.8102, -381.0732)
  line L182 (314.8102, -381.0732) -> (314.8102, -383.1377)
  line L183 (314.8102, -383.1377) -> (321.0537, -383.1377)
  line L184 (321.0537, -383.1377) -> (321.0537, -385.7902)
  line L185 (321.0537, -385.7902) -> (314.8102, -385.7902)
  line L186 (314.8102, -385.7902) -> (314.8102, -388.3552)
  line L187 (314.8102, -388.3552) -> (321.7419, -388.3552)
  line L188 (321.7419, -388.3552) -> (321.7419, -391.2955)
  line L189 (321.7419, -391.2955) -> (310.7813, -391.2955)
  line L190 (310.7813, -391.2955) -> (310.7813, -378.2955)
  line L191 (310.7813, -378.2955) -> (321.5417, -378.2955)
  line L192 (377.4204, -378.2955) -> (377.4204, -382.8499)
  line L193 (377.4204, -382.8499) -> (381.8121, -382.8499)
  line L194 (381.8121, -382.8499) -> (381.8121, -378.2955)
  line L195 (381.8121, -378.2955) -> (385.8535, -378.2955)
  line L196 (385.8535, -378.2955) -> (385.8535, -391.2955)
  line L197 (385.8535, -391.2955) -> (381.8121, -391.2955)
  line L198 (381.8121, -391.2955) -> (381.8121, -386.0405)
  line L199 (381.8121, -386.0405) -> (377.4204, -386.0405)
  line L200 (377.4204, -386.0405) -> (377.4204, -391.2955)
  line L201 (377.4204, -391.2955) -> (373.404, -391.2955)
  line L202 (373.404, -391.2955) -> (373.404, -378.2955)
  line L203 (373.404, -378.2955) -> (377.4204, -378.2955)
  line L204 (428.0941, -378.2955) -> (428.0941, -381.5111)
  line L205 (428.0941, -381.5111) -> (423.9902, -381.5111)
  line L206 (423.9902, -381.5111) -> (423.9902, -391.2955)
  line L207 (423.9902, -391.2955) -> (419.9738, -391.2955)
  line L208 (419.9738, -391.2955) -> (419.9738, -381.5111)
  line L209 (419.9738, -381.5111) -> (415.8699, -381.5111)
  line L210 (415.8699, -381.5111) -> (415.8699, -378.2955)
  line L211 (415.8699, -378.2955) -> (428.0941, -378.2955)
  line L212 (171.8364, -220.7379) -> (174.8364, -220.7379)
  line L213 (173.3364, -220.7379) -> (173.3364, -236.2379) construction
  circle A63 centre (173.3364, -220.7379) radius 1.5
  line L214 (177.3364, -220.7379) -> (177.3364, -234.2379)
  line L215 (175.3364, -236.2379) -> (171.3364, -236.2379)
  line L216 (169.3364, -234.2379) -> (169.3364, -220.7379)
  line L217 (173.3364, -217.3893) -> (176.2364, -219.0636)
  line L218 (176.2364, -219.0636) -> (176.2364, -222.4122)
  line L219 (176.2364, -222.4122) -> (173.3364, -224.0865)
  line L220 (173.3364, -224.0865) -> (170.4364, -222.4122)
  line L221 (170.4364, -222.4122) -> (170.4364, -219.0636)
  line L222 (170.4364, -219.0636) -> (173.3364, -217.3893)
  arc A64 (169.3364, -234.2379) -> (171.3364, -236.2379) centre (171.3364, -234.2379) ccw
  arc A65 (175.3364, -236.2379) -> (177.3364, -234.2379) centre (175.3364, -234.2379) ccw
  line L223 (171.8364, -227.7379) -> (174.8364, -227.7379)
  arc A66 (177.3364, -220.7379) -> (169.3364, -220.7379) centre (173.3364, -220.7379) ccw
  point P0 (0, 0)
  point P1 (218.1029, -306.1501)
  point P2 (217.7711, -306.0189)
  point P3 (217.438, -305.918)
  point P4 (217.1025, -305.8465)
  point P5 (216.1317, -305.8111)
  point P6 (220.4641, -309.7454)
  point P7 (220.3589, -309.0629)
  point P8 (220.1899, -308.4523)
  point P9 (219.961, -307.9077)
  point P10 (219.674, -307.4272)
  point P11 (219.3262, -307.0038)
  point P12 (218.9146, -306.6332)
  point P13 (221.8691, -304.7083)
  point P14 (222.4809, -305.2967)
  point P15 (223.0203, -305.9674)
  point P16 (223.4883, -306.7242)
  point P17 (223.863, -307.5474)
  point P18 (224.1368, -308.4504)
  point P19 (224.3064, -309.442)
  point P20 (220.6009, -317.1173)
  point P21 (220.0426, -317.3543)
  point P22 (219.456, -317.5399)
  point P23 (218.8392, -317.6742)
  point P24 (217.3279, -317.9034)
  point P25 (224.3057, -311.5794)
  point P26 (224.1289, -312.5529)
  point P27 (223.8391, -313.4597)
  point P28 (223.4349, -314.3113)
  point P29 (222.9364, -315.0982)
  point P30 (222.3869, -315.7748)
  point P31 (221.7863, -316.3492)
  point P32 (216.2639, -315.1052)
  point P33 (217.2603, -315.006)
  point P34 (217.6163, -314.9602)
  point P35 (217.9599, -314.8826)
  point P36 (218.2929, -314.7725)
  point P37 (219.038, -314.3186)
  point P38 (219.4058, -313.9592)
  point P39 (219.7231, -313.5468)
  point P40 (219.9911, -313.0769)
  point P41 (220.2062, -312.5477)
  point P42 (220.3657, -311.9482)
  point P43 (220.4657, -311.2705)
  point P44 (211.6384, -289.448)
  point P45 (211.8223, -289.5166)
  point P46 (211.9931, -289.5844)
  point P47 (212.1533, -289.6511)
  point P48 (212.3039, -289.7167)
  point P49 (212.4448, -289.7815)
  point P50 (212.5747, -289.846)
  point P51 (207.6179, -311.1953)
  point P52 (207.8112, -311.428)
  point P53 (207.9891, -311.6936)
  point P54 (208.1501, -311.9926)
  point P55 (208.2788, -312.3081)
  point P56 (208.3737, -312.6575)
  point P57 (208.4331, -313.0445)
  point P58 (208.0176, -307.0744)
  point P59 (207.8765, -307.6459)
  point P60 (207.6439, -308.1814)
  point P61 (207.3173, -308.6866)
  point P62 (206.9167, -309.1302)
  point P63 (206.4621, -309.4863)
  point P64 (205.9482, -309.7589)
  point P65 (206.8959, -303.8699)
  point P66 (207.2045, -304.1529)
  point P67 (207.4637, -304.4645)
  point P68 (207.6765, -304.8068)
  point P69 (207.8448, -305.1804)
  point P70 (207.9662, -305.5782)
  point P71 (208.0403, -306.0034)
  point P72 (205.9082, -310.2287)
  point P73 (206.4333, -310.4218)
  point P74 (206.6742, -310.5231)
  point P75 (206.9167, -310.6506)
  point P76 (207.1615, -310.8065)
  point P77 (204.2707, -306.864)
  point P78 (204.2301, -306.6678)
  point P79 (204.1659, -306.4987)
  point P80 (204.0783, -306.3519)
  point P81 (203.964, -306.2128)
  point P82 (203.8391, -306.0917)
  point P83 (203.7032, -305.9877)
  point P84 (203.3869, -305.8294)
  point P85 (203.2016, -305.7688)
  point P86 (202.9984, -305.7189)
  point P87 (202.7763, -305.6803)
  point P88 (202.2712, -305.6181)
  point P89 (203.8669, -302.7727)
  point P90 (204.9426, -302.9589)
  point P91 (205.8214, -303.2446)
  point P92 (201.343, -305.6269)
  point P93 (200.7841, -305.7185)
  point P94 (200.2001, -305.8682)
  point P95 (200.3105, -305.5758)
  point P96 (200.9732, -305.1178)
  point P97 (198.6349, -303.3503)
  point P98 (199.8644, -303.0256)
  point P99 (201.1826, -302.7926)
  point P100 (217.2894, -303.0746)
  point P101 (218.7692, -303.2383)
  point P102 (219.3919, -303.3879)
  point P103 (220.0002, -303.5965)
  point P104 (220.5961, -303.8658)
  point P105 (208.4269, -314.0291)
  point P106 (208.3471, -314.5509)
  point P107 (208.2169, -315.0416)
  point P108 (208.037, -315.504)
  point P109 (207.8102, -315.9336)
  point P110 (207.538, -316.3285)
  point P111 (207.2187, -316.6909)
  point P112 (206.0386, -289.8991)
  point P113 (206.196, -289.8709)
  point P114 (206.3528, -289.8271)
  point P115 (206.5085, -289.7683)
  point P116 (206.6634, -289.6947)
  point P117 (206.8184, -289.606)
  point P118 (206.9749, -289.5012)
  point P119 (207.716, -289.6221)
  point P120 (208.2579, -289.7859)
  point P121 (208.7773, -289.8807)
  point P122 (209.2865, -289.9118)
  point P123 (209.7957, -289.8807)
  point P124 (210.3151, -289.7859)
  point P125 (210.8571, -289.6221)
  point P126 (206.7023, -288.9995)
  point P127 (206.419, -289.1476)
  point P128 (206.165, -289.2242)
  point P129 (205.9237, -289.2508)
  point P130 (205.6808, -289.2317)
  point P131 (205.4217, -289.1579)
  point P132 (205.1305, -289.0065)
  point P133 (210.8913, -289.0415)
  point P134 (210.3208, -289.2354)
  point P135 (209.7945, -289.3434)
  point P136 (209.2887, -289.3781)
  point P137 (208.7827, -289.3434)
  point P138 (208.2555, -289.2354)
  point P139 (207.6837, -289.0414)
  point P140 (213.574, -288.7783)
  point P141 (213.4035, -288.7141)
  point P142 (213.2433, -288.6066)
  point P143 (213.0673, -288.4971)
  point P144 (212.8453, -288.4245)
  point P145 (212.5405, -288.4298)
  point P146 (212.1143, -288.5396)
  point P147 (441.0192, -389.2837)
  point P148 (441.3317, -389.1832)
  point P149 (441.6141, -389.0176)
  point P150 (441.8713, -388.782)
  point P151 (442.0864, -388.4822)
  point P152 (442.2498, -388.1029)
  point P153 (442.3561, -387.6285)
  point P154 (283.6156, -378.1425)
  point P155 (284.7701, -378.3317)
  point P156 (285.5686, -378.6146)
  point P157 (286.2413, -379.0048)
  point P158 (286.8189, -379.5036)
  point P159 (287.3105, -380.1197)
  point P160 (287.717, -380.8628)
  point P161 (284.0116, -382.1043)
  point P162 (283.8282, -381.8079)
  point P163 (283.6065, -381.5545)
  point P164 (283.3453, -381.3402)
  point P165 (283.0464, -381.1675)
  point P166 (282.7065, -381.0384)
  point P167 (282.3195, -380.9554)
  point P168 (286.4608, -390.4641)
  point P169 (285.0539, -391.0233)
  point P170 (283.6086, -391.3361)
  point P171 (282.6539, -388.5992)
  point P172 (283.2495, -388.5124)
  point P173 (283.8828, -388.3072)
  point P174 (275.0192, -383.7158)
  point P175 (275.1934, -382.7394)
  point P176 (275.4761, -381.8505)
  point P177 (275.8641, -381.041)
  point P178 (276.3496, -380.3221)
  point P179 (276.9317, -379.6948)
  point P180 (277.6164, -379.1534)
  point P181 (279.086, -378.4364)
  point P182 (279.8924, -378.2397)
  point P183 (280.8473, -378.1144)
  point P184 (281.2589, -380.9806)
  point P185 (280.7193, -381.1449)
  point P186 (280.2455, -381.4124)
  point P187 (279.8281, -381.7879)
  point P188 (279.4852, -382.2718)
  point P189 (279.2224, -382.9064)
  point P190 (279.0507, -383.7225)
  point P191 (279.0511, -385.8396)
  point P192 (279.2241, -386.6876)
  point P193 (279.4869, -387.3324)
  point P194 (279.8299, -387.8133)
  point P195 (280.2523, -388.1808)
  point P196 (280.7463, -388.4458)
  point P197 (281.3246, -388.6104)
  point P198 (280.1002, -391.3967)
  point P199 (278.7312, -391.0488)
  dimension "d0" = 3
  dimension "d1" = 7
  dimension "d3" = 5.8
  dimension "d4" = 2
  constraints: 436 end point, 98 point on circle, 59 centre point, 3 coincident, 2 midpoint, 1 point on line, 745 other
  measures "d0" diameter of A63
  measures "d1" distance from line of L15 L213.start
  measures "d3" distance between parallel lines of L218 L221
  measures "d4" radius of A64